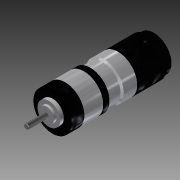
# Autodesk Inventor part: 14-0001
Saved by Autodesk Inventor 2015 SP1 (Build 190203100, 203)
## iProperties
Category: Standard Motor Kit
Company: Autodesk Inc.
Created: 2014-12-02
Part Number: 14-0001
Material: Generic
Document SubType Name: Modeling
Designer: Matrix
Density: 1 g/cm^3
Appearance: Default
Catalog Web Link: http://matrixrobotics.com/
Vendor: Matrix
Mass: 58.147 g
Surface Area: 98.8226 cm^2
Volume: 58.147 cm^3
Author: Autodesk Inc.
Autodesk Inventor part; units mm, degrees
ref_plane "YZ Plane" through (0, 0, 0) normal (1, 0, 0) x (0, 1, 0)
sketch "Sketch1" plane through (0, 0, 0) normal (0, 1, 0) x (-1, 0, 0)
  circle A0 centre (173.9561, -439.4442) radius 14
  dimension "d17" = 28
  constraints: 1 centre point
  measures "d17" diameter of A0
extrude "Extrusion1" add sketch "Sketch1" against normal blind 10
sketch "Sketch2" plane through (-173.9561, -10, -439.4442) normal (0, -1, 0) x (1, 0, 0)
  circle A0 centre (0, 0) radius 15.25
  point P0 (173.9561, 439.4442)
  dimension "d20" = 30.5
  constraints: 1 centre point
  measures "d20" diameter of A0
extrude "Extrusion2" add sketch "Sketch2" along normal blind 12
chamfer "Chamfer1" distance 1.25 angle 45 1 edges at (-189.2061, -10, -439.4442)
sketch "Sketch4" plane through (-173.9561, -22, -439.4442) normal (0, -1, 0) x (1, 0, 0)
  circle A0 centre (0, 0) radius 14
  point P0 (173.9561, 439.4442)
  dimension "d26" = 28
  constraints: 1 centre point
  measures "d26" diameter of A0
extrude "Extrusion3" add sketch "Sketch4" along normal blind 0.5
sketch "Sketch5" plane through (-173.9561, -22.5, -439.4442) normal (0, -1, 0) x (1, 0, 0)
  circle A0 centre (0, 0) radius 15.25
  point P0 (173.9561, 439.4442)
  dimension "d29" = 30.5
  constraints: 1 centre point
  measures "d29" diameter of A0
extrude "Extrusion4" add sketch "Sketch5" along normal blind 23
sketch "Sketch6" plane through (-173.9561, -45.5, -439.4442) normal (0, -1, 0) x (1, 0, 0)
  circle A0 centre (0, 0) radius 14
  point P0 (173.9561, 439.4442)
  dimension "d32" = 28
  constraints: 1 centre point
  measures "d32" diameter of A0
extrude "Extrusion5" add sketch "Sketch6" along normal blind 5
sketch "Sketch7" plane through (-173.9561, 0, -439.4442) normal (0, 1, 0) x (1, 0, 0)
  circle A0 centre (0, 0) radius 15.25
  point P0 (173.9561, -439.4442)
  dimension "d35" = 30.5
  constraints: 1 centre point
  measures "d35" diameter of A0
extrude "Extrusion6" add sketch "Sketch7" along normal blind 30
sketch "Sketch8" plane through (-173.9561, 30, -439.4442) normal (0, 1, 0) x (1, 0, 0)
  circle A0 centre (0, 0) radius 9
  point P0 (173.9561, -439.4442)
  dimension "d38" = 18
  constraints: 1 centre point
  measures "d38" diameter of A0
extrude "Extrusion7" add sketch "Sketch8" along normal blind 3
sketch "Sketch10" plane through (-173.9561, 33, -439.4442) normal (0, 1, 0) x (1, 0, 0)
  circle A0 centre (0, 0) radius 6.0592
  point P0 (173.9561, -439.4442)
  constraints: 1 centre point
extrude "Extrusion9" add sketch "Sketch10" along normal blind 2
sketch "Sketch11" plane through (-173.9561, 35, -439.4442) normal (0, 1, 0) x (1, 0, 0)
  circle A0 centre (0, 0) radius 2
  point P0 (173.9561, -439.4442)
  dimension "d45" = 4
  constraints: 1 centre point
  measures "d45" diameter of A0
extrude "Extrusion10" add sketch "Sketch11" along normal blind 16
fillet "Fillet1" radius 0.5 1 edges at (-175.9561, 51, -439.4442)
sketch "Sketch12" plane through (-173.9561, 51, -439.4442) normal (0, 1, 0) x (1, 0, 0)
  circle A0 centre (0, 0) radius 2 projected
  circle A1 centre (0, 0) radius 2 projected
  line L0 (-1.75, -0.9682) -> (-1.75, 0.9682)
  line L1 (1.75, -0.9682) -> (1.75, 0.9682)
  point P0 (173.9561, -439.4442)
  dimension "d49" = 3.5
  dimension "d50" = 1.75
  constraints: 8 point on circle, 4 end point, 2 vertical
  measures "d49" distance between parallel lines of L1 L0
  measures "d50" distance from line of A0.centre L0
extrude "Extrusion11" cut sketch "Sketch12" against normal blind 14 contours A0 L1 | L0 A0
ref_plane "Work Plane1" through (-173.9561, 20, -439.4442) normal (0, 1, 0) x (1, 0, 0)
ref_plane "Work Plane2" through (-173.9561, 5, -439.4442) normal (0, -1, 0) x (1, 0, 0)
split_face "Split1"
split_face "Split2"
equation "\"d50\" = 0.5 * d49"
body "Solid1"
